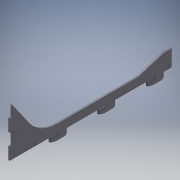
# Autodesk Inventor part: Camera mounting side
Saved by Autodesk Inventor 2017 (Build 210142000, 142)
## iProperties
Created: 2016-08-03
Part Number: Camera mounting side
Material: Generic
Document SubType Name: Modeling
Designer: Ali
Density: 1 g/cm^3
Appearance: Default
Author: Ali
Autodesk Inventor part; units mm, degrees
ref_plane "YZ Plane" through (0, 0, 0) normal (1, 0, 0) x (0, 1, 0)
ref_plane "XZ Plane" through (0, 0, 0) normal (0, 1, 0) x (-1, 0, 0)
ref_plane "XY Plane" through (0, 0, 0) normal (0, 0, 1) x (1, 0, 0)
sketch "Sketch1" plane through (0, 0, 0) normal (1, 0, 0) x (0, 1, 0)
  line L0 (0, 90) -> (0, 60)
  line L1 (400, 0) -> (400, 40)
  line L2 (6, 90) -> (0, 90)
  line L3 (360, 0) -> (360, -3)
  line L4 (353, -15) -> (375, -15)
  line L5 (380, -10) -> (380, 0)
  line L6 (353, -15) -> (340, -15) construction
  line L7 (340, -15) -> (340, -11) construction
  line L8 (340, -3) -> (360, -3)
  line L9 (0, 0) -> (360, 0)
  line L10 (380, 0) -> (400, 0)
  line L11 (340, -11) -> (353, -15)
  arc A0 (375, -15) -> (380, -10) centre (375, -10) ccw
  line L12 (340, -11) -> (340, -3)
  line L13 (240, 0) -> (240, -3)
  line L14 (220, -3) -> (240, -3)
  line L15 (220, -11) -> (220, -3)
  line L16 (260, -10) -> (260, 0)
  line L17 (233, -15) -> (255, -15)
  line L18 (233, -15) -> (220, -15) construction
  line L19 (220, -15) -> (220, -11) construction
  line L20 (220, -11) -> (233, -15)
  arc A1 (255, -15) -> (260, -10) centre (255, -10) ccw
  line L21 (120, 0) -> (120, -3)
  line L22 (100, -3) -> (120, -3)
  line L23 (100, -11) -> (100, -3)
  line L24 (140, -10) -> (140, 0)
  line L25 (113, -15) -> (135, -15)
  line L26 (113, -15) -> (100, -15) construction
  line L27 (100, -15) -> (100, -11) construction
  line L28 (100, -11) -> (113, -15)
  arc A2 (135, -15) -> (140, -10) centre (135, -10) ccw
  line L29 (240, 0) -> (260, 0)
  line L30 (120, 0) -> (140, 0)
  line L31 (6, 90) -> (6, 60) construction
  line L32 (0, 60) -> (6, 60)
  line L33 (6, 30) -> (0, 30)
  line L34 (0, 60) -> (0, 30) construction
  line L35 (0, 30) -> (0, 0)
  line L36 (6, 30) -> (6, 0) construction
  line L37 (6, 60) -> (6, 30)
  line L38 (400, 40) -> (380, 40)
  line L39 (380, 40) -> (316.8572, 20)
  line L40 (316.8572, 20) -> (116.5169, 20)
  line L41 (48.9774, 55) -> (6, 115.8967)
  arc A3 (48.9774, 55) -> (116.5169, 20) centre (116.5169, 102.6656) ccw
  line L42 (6, 90) -> (6, 115.8967)
  point P0 (24.2764, 90)
  dimension "d0" = 400
  dimension "d2" = 40
  dimension "d3" = 90
  dimension "d7" = 3
  dimension "d8" = 20
  dimension "d9" = 20
  dimension "d10" = 12
  dimension "d11" = 5
  dimension "d14" = 120
  dimension "d19" = 8
  dimension "d20" = 22
  dimension "d21" = 20
  dimension "d22" = 6
  dimension "d23" = 30
  dimension "d24" = 30
  constraints: 86 end point, 22 perpendicular, 8 point on circle, 5 parallel, 5 point on line, 4 centre point, 4 tangent, 4 vertical, 3 horizontal, 1 collinear, 38 other
  measures "d0" distance of L9.start L1.start
  measures "d2" distance of L1.start L1.end
  measures "d3" distance of L0.start L9.start
  measures "d7" distance between parallel lines of L8 L9
  measures "d8" distance between parallel lines of L5 L3
  measures "d9" distance of L8.start L3.end
  measures "d10" distance of L6.end L8.start
  measures "d11" radius of A0
  measures "d14" distance of L8.start L14.start
  measures "d19" distance of L7.end L8.start
  measures "d20" distance of L4.start L4.end
  measures "d21" distance between parallel lines of L5 L1
  measures "d22" distance between parallel lines of L0 L31
  measures "d23" distance between parallel lines of L33 L32
  measures "d24" distance of L33.start L36.end
extrude "Extrusion1" add sketch "Sketch1" along normal blind 3
sketch "Sketch2" plane through (3, 0, 0) normal (1, 0, 0) x (0, 0, -1)
  line L0 (-52, 16) -> (-36, 16) construction
  line L1 (-30, 0) -> (0, 0) projected
  line L2 (-30, 390) -> (-10, 390) construction
  line L3 (0, 400) -> (-40, 400) projected
  line L4 (0, 380) -> (0, 400) projected
  line L5 (0, 0) -> (0, 120) projected
  dimension "d25" = 16
  dimension "d26" = 16
  dimension "d27" = 20
  dimension "d28" = 10
  dimension "d29" = 10
  dimension "d30" = 36
  constraints: 4 end point, 2 horizontal
  measures "d25" distance of L0.end L0.start
  measures "d26" distance between parallel lines of L1 L0
  measures "d27" distance of L2.end L2.start
  measures "d28" distance between parallel lines of L3 L2
  measures "d29" distance from line of L4 L2.end
  measures "d30" distance from line of L5 L0.end
hole "Hole1" at (3, 16, 52) at (3, 16, 36) at (3, 390, 30) at (3, 390, 10) direction (-1, 0, 0) diameter 3.2 end through all
body "Solid1"
